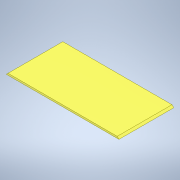
# Autodesk Inventor part: topForKetchenLight
Saved by Autodesk Inventor 2021.2 (Build 252289000, 289)
## iProperties
Created: 2021-02-17
Part Number: topForKetchenLight
Material: PC/ABS Plastic
Document SubType Name: Modeling
Designer: robst
Density: 0.357273 g/cm^3
Appearance: Smooth - Yellow
Author: robst
Autodesk Inventor part; units mm, degrees
ref_plane "YZ Plane" through (0, 0, 0) normal (1, 0, 0) x (0, 1, 0)
ref_plane "XZ Plane" through (0, 0, 0) normal (0, 1, 0) x (-1, 0, 0)
ref_plane "XY Plane" through (0, 0, 0) normal (0, 0, 1) x (1, 0, 0)
sketch "Sketch2" plane through (0, 0, 0) normal (0, 1, 0) x (-1, 0, 0)
  line L0 (101.6, 49.3535) -> (-101.6, 49.3535)
  line L1 (-101.6, 49.3535) -> (-101.6, -49.3535)
  line L2 (-101.6, -49.3535) -> (101.6, -49.3535)
  line L3 (101.6, -49.3535) -> (101.6, 49.3535)
  line L4 (101.6, 49.3535) -> (-101.6, -49.3535) construction
  line L5 (-101.6, 49.3535) -> (101.6, -49.3535) construction
  point P0 (0, 0)
  dimension "d0" = 98.7069
  dimension "d1" = 203.2
  constraints: 12 end point, 2 midpoint, 2 parallel, 1 horizontal, 1 perpendicular
  measures "d0" distance of L2.end L0.start
  measures "d1" distance of L1.end L2.end
extrude "Extrusion1" add sketch "Sketch2" along normal blind 3.175
sketch "Sketch3" plane through (-101.6, 0, 49.3535) normal (0, 0, 1) x (1, 0, 0)
  line L0 (0, 0) -> (0, 3.175) projected
  line L1 (0, 3.175) -> (203.2, 3.175) projected
  line L2 (0, 0) -> (203.2, 0) projected
  line L3 (203.2, 0) -> (0, 0) projected
  line L4 (0, 0) -> (3.175, 3.175)
  line L5 (203.2, 3.175) -> (0, 3.175) projected
  line L6 (3.175, 3.175) -> (0, 3.175)
  line L7 (0, 0) -> (0, 3.175) projected
  line L8 (0, 3.175) -> (0, 0)
  line L9 (203.2, 0) -> (203.2, 3.175) projected
  line L10 (203.2, 0) -> (200.025, 3.175)
  line L11 (200.025, 3.175) -> (203.2, 3.175)
  line L12 (203.2, 0) -> (203.2, 3.175) projected
  line L13 (203.2, 3.175) -> (203.2, 0)
  point P0 (101.6, 0)
  dimension "d4" = 45
  dimension "d5" = 45
  constraints: 12 end point, 3 collinear, 2 point on line, 1 vertical
  measures "d4" angle of L4 L2
  measures "d5" angle of L10 L2
extrude "Extrusion2" cut sketch "Sketch3" against normal through all contours L0 L1 L4 | L10 L1 L9
equation "\"d0\" = depth"
equation "\"d1\" = widthOfTop"
equation "\"d2\" = thickness"
equation "\"widthOfLightBracket\" = 285.75"
equation "\"depth\" = 98.70694"
equation "\"thickness\" = 3.175"
equation "\"widthOfTop\" = 203.2"
body "Solid1"
